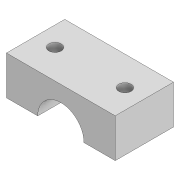
# Autodesk Inventor part: Landing_leg_rod_simulator_clamp_p2
Saved by Autodesk Inventor 2022 (Build 260153000, 153)
## iProperties
Created: 2022-04-29
Part Number: Landing_leg_rod_simulator_clamp_p2
Material: Generic
Document SubType Name: Modeling
Designer: dell
Density: 1 g/cm^3
Appearance: Default
Author: dell
Autodesk Inventor part; units mm, degrees
ref_plane "YZ Plane" through (0, 0, 0) normal (1, 0, 0) x (0, 1, 0)
ref_plane "XZ Plane" through (0, 0, 0) normal (0, 1, 0) x (-1, 0, 0)
ref_plane "XY Plane" through (0, 0, 0) normal (0, 0, 1) x (1, 0, 0)
sketch "Sketch1" plane through (0, 0, 0) normal (0, 0, 1) x (1, 0, 0)
  circle A0 centre (0, 0) radius 5.95
  line L0 (-14, 10) -> (14, 10)
  line L1 (14, 10) -> (14, -18)
  line L2 (14, -18) -> (-14, -18)
  line L3 (-14, -18) -> (-14, 10)
  dimension "d0" = 11.9
  dimension "d1" = 10
  dimension "d2" = 14
  dimension "d3" = 14
  dimension "d4" = 18
  constraints: 8 end point, 2 parallel, 1 centre point, 1 coincident, 1 horizontal, 1 perpendicular
  measures "d0" diameter of A0
  measures "d1" distance from line of L0 point (0, 0)
  measures "d2" distance from line of point (0, 0) L1
  measures "d3" distance from line of L3 A0.centre
  measures "d4" distance from line of L2 point (0, 0)
extrude "Extrusion1" add sketch "Sketch1" against normal blind 15
sketch "Sketch2" plane through (-14, -18, 0) normal (0, -1, 0) x (1, 0, 0)
  circle A0 centre (14, -7.5) radius 4.1
  line L0 (0, 0) -> (0, -15) projected
  line L1 (0, 0) -> (28, 0) projected
  point P0 (14, 0)
  dimension "d7" = 8.2
  dimension "d8" = 14
  dimension "d9" = 7.5
  constraints: 1 centre point
  measures "d7" diameter of A0
  measures "d8" distance from line of L0 A0.centre
  measures "d9" distance from line of L1 A0.centre
extrude "Extrusion2" cut sketch "Sketch2" against normal blind 10
sketch "Sketch3" plane through (-14, -18, 0) normal (0, -1, 0) x (1, 0, 0)
  circle A0 centre (23, -7.5) radius 1.6
  circle A1 centre (5, -7.5) radius 1.6
  line L0 (0, 0) -> (0, -15) projected
  line L1 (28, 0) -> (28, -15) projected
  line L2 (0, 0) -> (28, 0) projected
  point P0 (14, 0)
  dimension "d12" = 3.2
  dimension "d13" = 3.2
  dimension "d14" = 5
  dimension "d15" = 5
  dimension "d16" = 7.5
  dimension "d17" = 7.5
  constraints: 2 centre point
  measures "d12" diameter of A0
  measures "d13" diameter of A1
  measures "d14" distance from line of L0 A1.centre
  measures "d15" distance from line of L1 A0.centre
  measures "d16" distance from line of L2 A1.centre
  measures "d17" distance from line of L2 A0.centre
extrude "Extrusion3" cut sketch "Sketch3" against normal blind 100
sketch "Sketch4" plane through (0, 0, 0) normal (0, 1, 0) x (-1, 0, 0)
  line L0 (48.4223, 23.219) -> (-43.1506, 23.219)
  line L1 (-43.1506, 23.219) -> (-43.1506, -23.0413)
  line L2 (-43.1506, -23.0413) -> (48.4223, -23.0413)
  line L3 (48.4223, -23.0413) -> (48.4223, 23.219)
  point P0 (0, 0)
  constraints: 8 end point, 2 parallel, 1 horizontal, 1 perpendicular
extrude "Extrusion4" cut sketch "Sketch4" against normal blind 100
body "Solid1"
